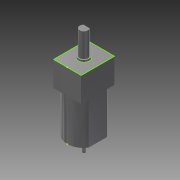
# Autodesk Inventor part: Motors
Saved by Autodesk Inventor 2015 (Build 190159000, 159)
## iProperties
Created: 2014-10-28
Part Number: Motors
Material: Stainless Steel
Document SubType Name: Modeling
Designer: s4201025
Density: 8.08 g/cm^3
Appearance: Semi-Polished
Author: s4201025
Autodesk Inventor part; units mm, degrees
ref_plane "YZ Plane" through (0, 0, 0) normal (1, 0, 0) x (0, 1, 0)
ref_plane "XZ Plane" through (0, 0, 0) normal (0, 1, 0) x (-1, 0, 0)
ref_plane "XY Plane" through (0, 0, 0) normal (0, 0, 1) x (1, 0, 0)
sketch "Sketch1" plane through (0, 0, 0) normal (0, 0, 1) x (1, 0, 0)
  line L0 (-5, 0) -> (5, 0)
  line L1 (5, 0) -> (5, 12)
  line L2 (5, 12) -> (-5, 12)
  line L3 (-5, 12) -> (-5, 0)
  arc A0 (-1.118, 7) -> (1.118, 7) centre (0, 6) ccw
  line L4 (0, 7) -> (-1.118, 7)
  line L5 (-1.118, 7) -> (1.118, 7)
  circle A1 centre (0, 6) radius 1.5
  circle A2 centre (0, 6) radius 1.95
  point P0 (0, 0)
  dimension "d0" = 10
  dimension "d1" = 12
  constraints: 12 end point, 3 centre point, 2 parallel, 2 point on circle, 1 horizontal, 1 perpendicular
  measures "d0" distance of L2.end L1.end
  measures "d1" distance of L1.end L0.end
extrude "Extrusion1" add sketch "Sketch1" along normal blind 9.271 contours L4 L5 A0
extrude "Extrusion2" add sketch "Sketch1" along normal blind 0.6 contours A2
extrude "Extrusion3" add sketch "Sketch1" along normal blind 0.6 contours A1 L5 L4
sketch "Sketch2" plane through (0, 6, 0) normal (0, 0, -1) x (-1, 0, 0)
  circle A0 centre (0, 0) radius 1.95 projected
  point P0 (0, -6)
extrude "Extrusion4" add sketch "Sketch1" against normal blind 9 contours L3 L2 L1 L0
extrude "Extrusion5" add sketch "Sketch2" along normal blind 9
sketch "Sketch4" plane through (0, 0, -9) normal (0, 0, -1) x (-1, 0, 0)
  line L0 (5, 9.3166) -> (5, 2.6834)
  line L1 (-5, 2.6834) -> (-5, 9.3166)
  arc A0 (5, 9.3166) -> (-5, 9.3166) centre (0, 6) ccw
  arc A1 (-5, 2.6834) -> (5, 2.6834) centre (0, 6) ccw
  point P0 (0, 0)
  constraints: 4 end point, 4 point on circle, 2 centre point, 1 parallel
extrude "Extrusion6" add sketch "Sketch4" along normal blind 15
sketch "Sketch5" plane through (0, 0, -24) normal (0, 0, -1) x (-1, 0, 0)
  circle A0 centre (0, 6) radius 2.5
  circle A1 centre (0, 6) radius 0.5
  point P0 (0, 0)
  constraints: 2 centre point
extrude "Extrusion7" add sketch "Sketch5" along normal blind 1
extrude "Extrusion8" add sketch "Sketch5" along normal blind 5.5 contours A1
sketch "Sketch6" plane through (-5, 0, 0) normal (0, -1, 0) x (1, 0, 0)
  line L0 (0, 0) -> (10, 0) projected
  line L1 (0, 0) -> (0, -9) projected
  line L2 (5, -9) -> (0, -9) projected
  line L3 (10, -9) -> (5, -9) projected
  line L4 (10, 0) -> (10, -9) projected
  line L5 (5, -9) -> (10, -9) projected
  line L6 (0, -9) -> (5, -9) projected
  line L7 (0, -9) -> (0, -24) projected
  line L8 (10, -24) -> (0, -24) projected
  line L9 (10, -9) -> (10, -24) projected
  line L10 (0, 0) -> (10, 0) projected
  line L11 (0, 0) -> (0, -9) projected
  line L12 (5, -9) -> (0, -9) projected
  line L13 (10, -9) -> (5, -9) projected
  line L14 (10, 0) -> (10, -9) projected
  line L15 (3.882, 0.6) -> (6.118, 0.6) projected
  line L16 (6.118, 0.6) -> (6.118, 9.271) projected
  line L17 (3.882, 9.271) -> (6.118, 9.271) projected
  line L18 (3.882, 0.6) -> (3.882, 9.271) projected
  line L19 (6.95, 0.6) -> (3.05, 0.6) projected
  line L20 (3.5, 0.6) -> (3.5, 9.271) projected
  line L21 (4.5, -29.5) -> (5.5, -29.5) projected
  line L22 (5.5, -25) -> (4.5, -25) projected
  line L23 (2.5, -25) -> (7.5, -25) projected
  line L24 (7.5, -24) -> (2.5, -24) projected
  line L25 (5.5, -25) -> (5.5, -29.5) projected
  line L26 (4.5, -25) -> (4.5, -29.5) projected
  line L27 (2.5, -24) -> (2.5, -25) projected
  line L28 (2.5, -25) -> (7.5, -25) projected
  line L29 (7.5, -24) -> (7.5, -25) projected
  line L30 (6.5, 0.6) -> (6.5, 9.271) projected
  line L31 (6.95, 0) -> (6.95, 0.6) projected
  line L32 (3.05, 0) -> (3.05, 0.6) projected
  line L33 (6.5, 9.271) -> (3.5, 9.271) projected
  point P0 (5, 0)
body "Solid1"
